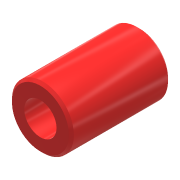
# Autodesk Inventor part: ARL-2608E
Saved by Autodesk Inventor 2018 (Build 220112000, 112)
## iProperties
Created: 2018-08-31
Part Number: ARL-2608E
Material: 一般
Document SubType Name: Modeling
Designer: student
Density: 1 g/cm^3
Appearance: 淡い赤
Author: student
Autodesk Inventor part; units mm, degrees
ref_plane "YZ Plane" through (0, 0, 0) normal (1, 0, 0) x (0, 1, 0)
ref_plane "XZ Plane" through (0, 0, 0) normal (0, 1, 0) x (-1, 0, 0)
ref_plane "XY Plane" through (0, 0, 0) normal (0, 0, 1) x (1, 0, 0)
sketch "スケッチ1" plane through (0, 0, 0) normal (0, 1, 0) x (1, 0, 0)
  circle A0 centre (0, 0) radius 2.5
  circle A1 centre (0, 0) radius 1.3
  dimension "d0" = 5
  dimension "d1" = 2.6
  constraints: 2 centre point, 2 coincident
  measures "d0" diameter of A0
  measures "d1" diameter of A1
extrude "押し出し1" add sketch "スケッチ1" along normal mid plane 8
chamfer "面取り1" distance 0.2 angle 45 2 edges at (-2.5, 4, 0) (-2.5, -4, 0)
